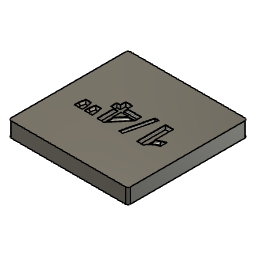
Magnet_Spacer _1-4 (Autodesk Fusion 360 design; units mm, degrees)
Autodesk Fusion 360 part; units mm, degrees
note: some values were not read from the file. Set by a fixed rule: which face or edge a step refers to.
sketch "Sketch1" plane through (0, 0, 0) normal (0, 1, 0) x (1, 0, 0)
  line L0 (0, -56.9323) -> (0, 40) construction
  line L1 (29.5824, 0) -> (-37.1077, 0) construction
  line L2 (12.7, -12.7) -> (-12.7, -12.7)
  line L3 (-12.7, -12.7) -> (-12.7, 12.7)
  line L4 (-12.7, 12.7) -> (12.7, 12.7)
  line L5 (12.7, 12.7) -> (12.7, -12.7)
  dimension "d1" = 25.4
  constraint vertical L0
  constraint perpendicular L0 L1
  constraint coincident origin L0
  constraint coincident origin L1
  constraint horizontal L2
  constraint vertical L3
  constraint horizontal L4
  constraint vertical L5
  constraint equal L2 L3
  constraint symmetric L0 L3 L5
  constraint symmetric L1 L2 L4
  measures "d1" distance of L2.start L2.end
extrude "Extrude1" add sketch "Sketch1" along normal blind 3.175
sketch "Sketch2" plane through (0, 3.175, 0) normal (0, 1, 0) x (-1, 0, 0)
  line L0 (-12.7, -12.7) -> (12.7, -12.7)
  line L1 (12.7, -12.7) -> (12.7, 12.7)
  line L2 (12.7, 12.7) -> (-12.7, 12.7)
  line L3 (-12.7, 12.7) -> (-12.7, -12.7)
  line L4 (-7.2802, -6.4414) -> (7.2802, -6.4414) construction
  line L5 (7.2802, -6.4414) -> (7.2802, 6.4414) construction
  line L6 (7.2802, 6.4414) -> (-7.2802, 6.4414) construction
  line L7 (-7.2802, 6.4414) -> (-7.2802, -6.4414) construction
  line L8 (0, 6.4414) -> (0, -6.4414) construction
  line L9 (-7.2802, 0) -> (7.2802, 0) construction
  point P0 (-7.2802, 6.4414)
  dimension "d6" = 6
  text T0 "1/4\"" font "Arial Black" height 6 bold align centre middle in box 14.5604 x 12.8827 at (-7.2802, -6.4414) x (1, 0) y (0, 1) spacing 1
  constraint coincident P0
  constraint midpoint L6 L8.start
  constraint midpoint L4 L8.end
  constraint midpoint L7 L9.start
  constraint midpoint L5 L9.end
  constraint symmetric L1 L3 L8
  constraint symmetric L0 L2 L9
extrude "Extrude2" cut sketch "Sketch2" against normal blind 0.5 text T0
fillet "Fillet1" radius 0.4 5 faces at (5.5327, 2.675, 0.367) (1.9338, 2.675, 1.0355) (-3.0048, 2.675, 1.2729) (-5.2585, 2.675, 1.6044) (-7.3909, 2.675, 1.6044)
fillet "Fillet2" radius 0.5 4 edges at (-12.7, 1.5875, 12.7) (12.7, 1.5875, 12.7) (12.7, 1.5875, -12.7) (-12.7, 1.5875, -12.7)
